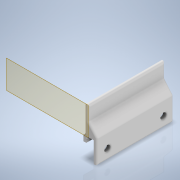
# Autodesk Inventor part: BackPistonSupportButtom
Saved by Autodesk Inventor 2022.2 (Build 262287000, 287)
## iProperties
Created: 2022-02-16
Part Number: BackPistonSupportButtom
Material: Generic
Document SubType Name: Modeling
Designer: siwat
Density: 1 g/cm^3
Appearance: Default
Author: siwat
Autodesk Inventor part; units mm, degrees
ref_plane "YZ Plane" through (0, 0, 0) normal (1, 0, 0) x (0, 1, 0)
ref_plane "XZ Plane" through (0, 0, 0) normal (0, 1, 0) x (-1, 0, 0)
ref_plane "XY Plane" through (0, 0, 0) normal (0, 0, 1) x (1, 0, 0)
ref_plane "Work Plane1" through (0, 0, 0) normal (0, 0, 1) x (1, 0, 0)
sketch "Sketch1" plane through (0, 0, 0) normal (0, 0, 1) x (1, 0, 0)
  line L0 (40.5785, -1.8781) -> (40.5785, -3.2427)
  line L1 (40.5785, -3.2427) -> (38.2445, -5.6804)
  line L2 (38.2445, -5.6804) -> (35.4492, -5.6804)
  line L3 (35.4492, -5.6804) -> (35.4492, -0.1275)
  line L4 (35.4492, -0.1275) -> (37.5785, -0.1275)
  line L5 (37.5785, -0.1275) -> (37.5785, 27.0272)
  line L6 (37.5785, 27.0272) -> (40.5785, 27.0272)
  line L7 (40.5785, 27.0272) -> (40.5785, 0.1566)
  line L8 (40.5785, 0.1566) -> (40.0286, 0.1566)
  line L9 (40.0286, 0.1566) -> (38.1588, -1.796)
  line L10 (38.1588, -1.796) -> (38.0803, -1.8781)
  line L11 (38.0803, -1.8781) -> (40.5785, -1.8781)
  line L12 (40.5785, 3.1566) -> (48.9527, 3.1566)
  line L13 (48.9527, 3.1566) -> (48.9527, -20.1251)
  line L14 (48.9527, -20.1251) -> (45.5698, -20.1251)
  line L15 (45.5698, -20.1251) -> (45.5698, 0.1566)
  line L16 (45.5698, 0.1566) -> (40.5785, 0.1566)
  point P0 (0, 0)
  dimension "d0" = 3
  dimension "d1" = 3
  dimension "d2" = 43.757
  dimension "d3" = 3.3829
  dimension "d4" = 8.3742
  dimension "d5" = 13.5035
  dimension "d6" = 23.2817
  dimension "d7" = 18.247
  dimension "d8" = 47.1522
  dimension "d9" = 14.4447
  dimension "d10" = 19.9975
  dimension "d11" = 2.7483
  dimension "d12" = 48.9527
  dimension "d13" = 20.1251
  dimension "d14" = 31.5517
  dimension "d15" = 10.7939
  constraints: 34 end point, 10 perpendicular, 4 point on line, 2 parallel, 1 horizontal, 1 vertical
  measures "d0" distance of L5.end L6.end
  measures "d1" distance between parallel lines of L12 L16
  measures "d2" angle of L1 L13
  measures "d3" distance between parallel lines of L15 L13
  measures "d4" distance between parallel lines of L0 L13
  measures "d5" distance between parallel lines of L3 L13
  measures "d6" distance between parallel lines of L12 L14
  measures "d7" distance between parallel lines of L11 L14
  measures "d8" distance between parallel lines of L14 L6
  measures "d9" distance between parallel lines of L2 L14
  measures "d10" distance between parallel lines of L4 L14
  measures "d11" distance between parallel lines of L9 L1
  measures "d12" distance from line of point (0, 0) L13
  measures "d13" distance from line of point (0, 0) L14
  measures "d14" distance from line of point (0, 0) L1
  measures "d15" distance from line of L9.end L13
extrude "Extrusion1" add sketch "Sketch1" against normal blind 75
draft "FaceDraft1" angle -50 pull direction (-1, 0, 0) faces at (46.1613, 3.1566, -25) fixed edges at (48.9527, 3.1566, -37.5)
sketch "Sketch2" plane through (48.9527, -20.1251, 0) normal (1, 0, 0) x (0, 0, -1)
  circle A0 centre (10, 10) radius 3
  circle A1 centre (65, 10) radius 3
  line L0 (10, 10) -> (65, 10)
  line L1 (0, 0) -> (0, 23.2817) projected
  line L2 (75, 23.2817) -> (75, 0) projected
  line L3 (0, 0) -> (75, 0) projected
  point P0 (0, 20.1251)
  dimension "d19" = 6
  dimension "d20" = 6
  dimension "d21" = 10
  dimension "d22" = 10
  dimension "d23" = 10
  constraints: 2 centre point, 2 end point, 1 horizontal
  measures "d19" diameter of A0
  measures "d20" diameter of A1
  measures "d21" distance from line of L0.start L1
  measures "d22" distance from line of L2 L0.end
  measures "d23" distance from line of L3 L0.start
extrude "Extrusion2" cut sketch "Sketch2" against normal through all
fillet "Fillet1" radius 2 11 edges at (48.9527, -8.4842, 0) (48.9527, -20.1251, -37.5) (48.9527, -8.4842, -75) (40.0286, 0.1566, -37.5) (40.5785, 13.1366, -37.5) (44.7656, 8.1466, 0) (44.7656, 8.1466, -75) (48.9527, 3.1566, -37.5) (40.5785, 20.0819, 0) (40.5785, 27.0272, -37.5) (40.5785, 20.0819, -75)
equation "\"d22\" = d21"
body "Solid1"
